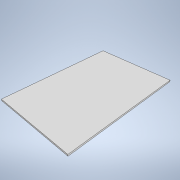
# Autodesk Inventor part: lower casing
Saved by Autodesk Inventor 2020 (Build 240168000, 168)
## iProperties
Created: 2019-06-23
Part Number: lower casing
Material: Generic
Document SubType Name: Modeling
Designer: jjsch
Density: 1 g/cm^3
Appearance: Default
Author: jjsch
Autodesk Inventor part; units mm, degrees
ref_plane "YZ Plane" through (0, 0, 0) normal (1, 0, 0) x (0, 1, 0)
ref_plane "XZ Plane" through (0, 0, 0) normal (0, 1, 0) x (-1, 0, 0)
ref_plane "XY Plane" through (0, 0, 0) normal (0, 0, 1) x (1, 0, 0)
sketch "Sketch1" plane through (0, 0, 0) normal (0, 1, 0) x (-1, 0, 0)
  line L0 (-56.5685, -84) -> (56.5685, -84)
  line L1 (56.5685, -84) -> (56.5685, 84)
  line L2 (56.5685, 84) -> (-56.5685, 84)
  line L3 (-56.5685, 84) -> (-56.5685, -84)
  line L4 (-56.5685, -84) -> (56.5685, 84) construction
  line L5 (56.5685, -84) -> (-56.5685, 84) construction
  point P0 (0, 0)
  dimension "d0" = 168
  dimension "d1" = 113.1371
  constraints: 12 end point, 2 midpoint, 2 parallel, 1 horizontal, 1 perpendicular
  measures "d0" distance of L1.end L0.end
  measures "d1" distance of L1.end L2.end
extrude "Extrusion1" add sketch "Sketch1" along normal blind 2.4
body "Solid1"
